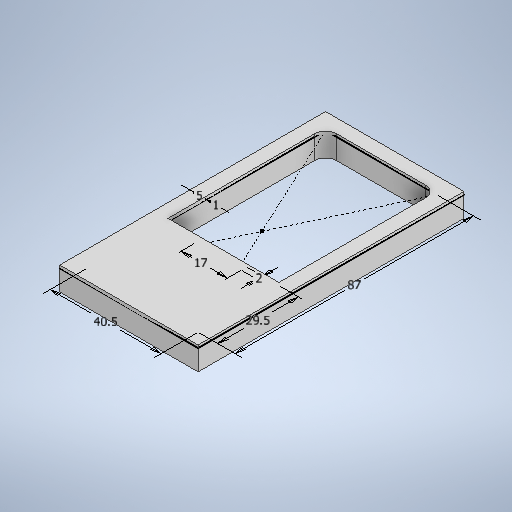
# Autodesk Inventor part: manija_puerta_marco_front_right_v2
Saved by Autodesk Inventor 2025.1 (Build 291241020, 241B)
## iProperties
Created: 2024-12-04
Part Number: manija_puerta_marco_front_right_v2
Material: Genérico
Document SubType Name: Modeling
Designer: ctamashiro
Density: 1 g/cm^3
Appearance: Valor por defecto
Author: ctamashiro
Autodesk Inventor part; units mm, degrees
ref_plane "YZ Plane" through (0, 0, 0) normal (1, 0, 0) x (0, 1, 0)
ref_plane "XZ Plane" through (0, 0, 0) normal (0, 1, 0) x (-1, 0, 0)
ref_plane "XY Plane" through (0, 0, 0) normal (0, 0, 1) x (1, 0, 0)
sketch "Boceto1" plane through (0, 0, 0) normal (0, 1, 0) x (-1, 0, 0)
  line L0 (20.25, -43.5) -> (-20.25, -43.5)
  line L1 (-20.25, -43.5) -> (-20.25, 43.5)
  line L2 (-20.25, 43.5) -> (20.25, 43.5)
  line L3 (20.25, 43.5) -> (20.25, -43.5)
  line L4 (20.25, -43.5) -> (-20.25, 43.5) construction
  line L5 (-20.25, -43.5) -> (20.25, 43.5) construction
  line L6 (25.25, -48.5) -> (-25.25, -48.5)
  line L7 (-25.25, -48.5) -> (-25.25, 48.5)
  line L8 (-25.25, 48.5) -> (25.25, 48.5)
  line L9 (25.25, 48.5) -> (25.25, -48.5)
  line L10 (20.25, 43.5) -> (-20.25, 43.5)
  line L11 (-20.25, 43.5) -> (-20.25, 14)
  line L12 (-20.25, 14) -> (20.25, 14)
  line L13 (20.25, 14) -> (20.25, 43.5)
  line L14 (25.25, 14) -> (-25.25, 14)
  line L15 (21.25, -44.5) -> (-21.25, -44.5)
  line L16 (-21.25, -44.5) -> (-21.25, 44.5)
  line L17 (-21.25, 44.5) -> (21.25, 44.5)
  line L18 (21.25, 44.5) -> (21.25, -44.5)
  line L19 (8.5, 14) -> (-8.5, 14)
  line L20 (-8.5, 14) -> (-8.5, 16)
  line L21 (-8.5, 16) -> (8.5, 16)
  line L22 (8.5, 16) -> (8.5, 14)
  point P0 (0, 0)
  point P1 (0, 0)
  point P2 (-20.25, 14)
  point P3 (20.25, 14)
  point P4 (-20.25, 14)
  point P5 (0, 14)
  dimension "d0" = 40.5
  dimension "d1" = 87
  dimension "d2" = 5
  dimension "d3" = 29.5
  dimension "d19" = 1
  dimension "d20" = 17
  dimension "d21" = 2
  constraints: 46 end point, 10 parallel, 5 perpendicular, 5 point on line, 4 midpoint, 3 horizontal, 1 coincident, 6 other
  measures "d0" distance of L1.end L2.end
  measures "d1" distance of L0.end L1.end
  measures "d2" distance between parallel lines of L3 L9
  measures "d3" distance of L11.end L10.end
  measures "d19" distance between parallel lines of L3 L18
  measures "d20" distance of L20.end L21.end
  measures "d21" distance between parallel lines of L21 L19
extrude "Extrusión4" add sketch "Boceto1" against normal blind 7.5 contours L3 L14 L18 L15 L16 L1 L0 | L3 L2 L1 L14 L16 L17 L18 | L18 L17 L16 L14 L7 L8 L9 | L14 L9 L6 L7 L16 L15 L18
extrude "Extrusión5" add sketch "Boceto1" along normal blind 1 contours L3 L14 L18 L15 L16 L1 L0 | L12 L22 L21 L20 L1 L2 L3 | L3 L2 L1 L14 L16 L17 L18 | L12 L20 L21 L22 | L18 L17 L16 L14 L7 L8 L9 | L14 L9 L6 L7 L16 L15 L18
fillet "Empalme2" radius 4 4 edges at (-20.25, -3.25, -43.5) (20.25, -3.25, -43.5) (20.25, -3.75, 43.5) (-20.25, -3.75, 43.5)
fillet "Empalme3" radius 2 1 edges at (0, 0, 14)
